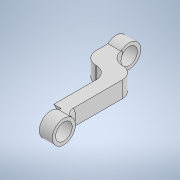
# Autodesk Inventor part: Рулевая тяга
Saved by Autodesk Inventor 2020 (Build 240168000, 168)
## iProperties
Created: 2021-07-18
Part Number: Рулевая тяга
Material: Типовые
Document SubType Name: Modeling
Designer: Антон
Density: 1 g/cm^3
Appearance: По умолчанию
Author: Антон
Autodesk Inventor part; units mm, degrees
ref_plane "YZ Plane" through (0, 0, 0) normal (1, 0, 0) x (0, 1, 0)
ref_plane "XZ Plane" through (0, 0, 0) normal (0, 1, 0) x (-1, 0, 0)
ref_plane "XY Plane" through (0, 0, 0) normal (0, 0, 1) x (1, 0, 0)
sketch "Эскиз1" plane through (0, 0, 0) normal (0, 1, 0) x (-1, 0, 0)
  line L0 (0, 0) -> (4, 0)
  line L1 (4, 0) -> (4, -23.9397)
  line L2 (4, -23.9397) -> (0, -23.9397)
  line L3 (0, -23.9397) -> (0, 0)
  line L4 (0, -23.9397) -> (11.75, -23.9397)
  line L5 (11.75, -23.9397) -> (11.75, -19.9397)
  line L6 (11.75, -19.9397) -> (0, -19.9397)
  line L7 (0, -19.9397) -> (0, -23.9397)
  line L8 (11.75, -19.9397) -> (7.75, -19.9397)
  line L9 (7.75, -19.9397) -> (7.75, -29.9397)
  line L10 (7.75, -29.9397) -> (11.75, -29.9397)
  line L11 (11.75, -29.9397) -> (11.75, -19.9397)
  line L12 (11.75, -23.9397) -> (4, -19.9397)
  line L13 (0, -19.9397) -> (7.75, -23.9397)
  point P0 (3, -20.536)
  point P1 (0, -19.9397)
  dimension "d10" = 4
  dimension "d11" = 11.75
  dimension "d36" = 29.9397
  dimension "d55" = 10
  constraints: 28 end point, 6 parallel, 4 point on line, 3 horizontal, 3 perpendicular, 2 equal length
  measures "d10" distance of L0.start L0.end
  measures "d11" distance between parallel lines of L3 L11
  measures "d36" distance between parallel lines of L10 L0
  measures "d55" distance of L10.end L5.end
extrude "Выдавливание1" add sketch "Эскиз1" along normal blind 5
fillet "Сопряжение2" radius 3.855 4 edges at (-4, 2.5, -19.9397) (-11.75, 2.5, -19.9397) (0, 2.5, -23.9397) (-7.75, 2.5, -23.9397)
sketch "Эскиз7" plane through (-11.75, 0, -29.9397) normal (-1, 0, 0) x (0, 0, 1)
  line L0 (0, 0) -> (0, 5) projected
  circle A0 centre (0, 2.5) radius 2.525
  circle A1 centre (0, 2.5) radius 3.525
  point P0 (29.9397, 0)
  point P1 (0, 4.975)
  point P2 (0, 0.025)
  dimension "d37" = 5.05
  dimension "d38" = 7.05
  constraints: 2 centre point, 1 coincident, 1 midpoint
  measures "d37" diameter of A0
  measures "d38" diameter of A1
extrude "Выдавливание5" add sketch "Эскиз7" against normal up to surface (4 mm away) contours A0 | A1
extrude "Выдавливание8" cut sketch "Эскиз7" against normal through all contours A0
sketch "Эскиз8" plane through (-4, 0, 0) normal (-1, 0, 0) x (0, 0, 1)
  line L0 (0, 0) -> (0, 5) projected
  circle A0 centre (0, 2.5) radius 2.525
  circle A1 centre (0, 2.5) radius 3.525
  point P0 (0, 4.975)
  point P1 (0, 0.025)
  dimension "d41" = 5.05
  dimension "d42" = 7.05
  constraints: 2 centre point, 1 coincident, 1 midpoint
  measures "d41" diameter of A0
  measures "d42" diameter of A1
extrude "Выдавливание6" add sketch "Эскиз8" against normal up to surface (4 mm away)
extrude "Выдавливание7" cut sketch "Эскиз8" against normal through all contours A0
sketch "Эскиз9" plane through (-4, 0, -20.0847) normal (1, 0, 0) x (0, 0, -1)
  circle A0 centre (-20.0847, 2.5) radius 2.525 projected
  circle A1 centre (-20.0847, 2.5) radius 4.025
  arc A2 (-17.5996, 5) -> (-17.5996, 0) centre (-20.0847, 2.5) ccw projected
  point P0 (-20.0847, 0)
  point P1 (-20.0847, 4.975)
  point P2 (-20.0847, 0.025)
  point P3 (-19.7302, 5)
  point P4 (-19.7302, 0)
  dimension "d49" = 0.5
  constraints: 1 centre point, 1 coincident
  measures "d49" radial gap between concentric circles of A1 A2
extrude "Выдавливание9" cut sketch "Эскиз9" along normal blind 2.25 contours A0 | A1
sketch "Эскиз10" plane through (0, 0, -16.0847) normal (-1, 0, 0) x (0, 0, 1)
  arc A0 (13.5996, 0) -> (13.5996, 5) centre (16.0847, 2.5) ccw projected
  circle A1 centre (16.0847, 2.5) radius 3.525
  circle A2 centre (16.0847, 2.5) radius 2.525 projected
  point P0 (12.3578, 0)
  point P1 (12.3578, 5)
  point P2 (13.5996, 5)
  point P3 (13.5996, 0)
  point P4 (13.671, 5)
  point P5 (13.671, 0)
  constraints: 1 centre point, 1 coincident, 1 concentric
extrude "Выдавливание10" add sketch "Эскиз10" against normal blind 2.25
fillet "Сопряжение6" radius 2.25 1 edges at (0, 2.5, -3.525)
